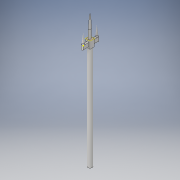
# Autodesk Inventor part: gungnir
Saved by Autodesk Inventor 2017 (Build 210142000, 142)
## iProperties
Created: 2016-12-22
Part Number: gungnir
Material: Generic
Document SubType Name: Modeling
Designer: theoren75306
Density: 1 g/cm^3
Appearance: Default
Author: theoren75306
Autodesk Inventor part; units mm, degrees
ref_plane "YZ Plane" through (0, 0, 0) normal (1, 0, 0) x (0, 1, 0)
ref_plane "XZ Plane" through (0, 0, 0) normal (0, 1, 0) x (-1, 0, 0)
ref_plane "XY Plane" through (0, 0, 0) normal (0, 0, 1) x (1, 0, 0)
sketch "Sketch1" plane through (0, 0, 0) normal (0, 1, 0) x (-1, 0, 0)
  circle A0 centre (0, 0) radius 38.1
  dimension "d0" = 76.2
  constraints: 1 centre point, 1 coincident
  measures "d0" diameter of A0
extrude "Extrusion1" add sketch "Sketch1" along normal blind 1828.8
sketch "Sketch2" plane through (0, 1828.8, 0) normal (0, 1, 0) x (1, 0, 0)
  circle A0 centre (0, 0) radius 38.1 projected
  line L0 (0, -38.1) -> (-38.1, -38.1)
  line L1 (-38.1, -38.1) -> (-38.1, 38.1)
  line L2 (-38.1, 38.1) -> (38.1, 38.1)
  line L3 (38.1, 38.1) -> (38.1, -38.1)
  line L4 (38.1, -38.1) -> (0, -38.1)
  constraints: 10 end point, 4 perpendicular, 3 horizontal, 1 point on line, 1 vertical alignment, 1 other
extrude "Extrusion2" add sketch "Sketch2" along normal blind 127 contours L0 L1 A0 | A0 L3 L4 | A0 L2 L3 | L1 L2 A0
ref_plane "Work Plane1" through (-26.9408, 1955.8, -26.9408) normal (0, 1, 0) x (1, 0, 0)
sketch "Sketch3" plane through (-26.9408, 1955.8, -26.9408) normal (0, 1, 0) x (1, 0, 0)
  circle A0 centre (26.9408, -26.9408) radius 38.1
  constraints: 1 centre point, 1 coincident
extrude "Extrusion3" add sketch "Sketch3" against normal blind 127
sketch "Sketch4" plane through (-38.1, 1828.8, 38.1) normal (0, 0, 1) x (1, 0, 0)
  line L0 (19.05, 32.3592) -> (57.15, 32.3592)
  line L1 (57.15, 32.3592) -> (57.15, 96.4699)
  line L2 (57.15, 96.4699) -> (19.05, 96.4699)
  line L3 (19.05, 96.4699) -> (19.05, 32.3592)
  arc A0 (19.05, 32.3592) -> (57.15, 32.3592) centre (38.1, 32.3592) ccw
  arc A1 (40.4667, 110.4399) -> (19.05, 96.4699) centre (53.0396, 67.7636) ccw
  arc A2 (57.15, 96.4699) -> (40.4667, 110.4399) centre (24.3533, 74.2501) ccw
  line L4 (0, 0) -> (0, 127) projected
  line L5 (76.2, 0) -> (76.2, 127) projected
  point P0 (38.1, -1828.8)
  dimension "d8" = 19.05
  dimension "d9" = 19.05
  dimension "d10" = 13.97
  constraints: 8 end point, 6 point on circle, 3 centre point, 2 parallel, 2 tangent, 1 horizontal, 1 perpendicular
  measures "d8" distance between parallel lines of L4 L3
  measures "d9" distance between parallel lines of L5 L1
  measures "d10" distance from line of L2 A1.start
extrude "Extrusion4" add sketch "Sketch4" along normal blind 101.6 contours L3 L2 L1 L0 | L0 A0
sketch "Sketch5" plane through (-38.1, 1828.8, 38.1) normal (0, 0, 1) x (1, 0, 0)
  line L0 (19.05, 32.3592) -> (19.05, 96.4699) projected
  arc A0 (38.1, 110.3729) -> (19.05, 96.4699) centre (49.9899, 74.0785) ccw
  arc A1 (56.8516, 96.4699) -> (38.1, 110.3729) centre (19.2002, 65.2848) ccw
  line L1 (19.05, 96.4699) -> (56.8516, 96.4699)
  line L2 (0, 127) -> (76.2, 127) projected
  point P0 (38.1, -1828.8)
  constraints: 4 point on circle, 2 centre point, 2 end point, 1 parallel
extrude "Extrusion5" add sketch "Sketch5" along normal blind 63.5
sketch "Sketch6" plane through (-19.05, 1925.2699, 139.7) normal (0, 1, 0) x (1, 0, 0)
  point P0 (19.05, 139.7)
sketch "Sketch7" plane through (-19.05, 1925.2699, 139.7) normal (0, 1, 0) x (1, 0, 0)
  point P0 (19.05, 139.7)
  point P1 (38.1, 0)
  point P2 (19.05, 38.1)
sketch "Sketch9" plane through (-19.05, 1925.2699, 139.7) normal (0, 1, 0) x (1, 0, 0)
  circle A0 centre (19.05, 19.0106) radius 19.05
  line L0 (38.1, 101.6) -> (38.1, 0) projected
  point P0 (19.05, 139.7)
  dimension "d25" = 38.1
  constraints: 1 centre point, 1 tangent
  measures "d25" diameter of A0
extrude "Extrusion6" add sketch "Sketch9" along normal blind 177.8
ref_plane "Work Plane4" through (38.1, 1828.8, 0) normal (0, 0, -1) x (-1, 0, 0)
mirror "Mirror1" about plane through (38.1, 1828.8, 0) normal (0, 0, -1) of "Extrusion4", "Extrusion5", "Extrusion6"
sketch "Sketch10" plane through (0, 1955.8, 0) normal (0, 1, 0) x (1, 0, 0)
  arc A0 (0, 28.3756) -> (0, -29.7598) centre (27.6643, -0.6921) ccw
  line L0 (0, -38.1) -> (-19.05, -38.1) projected
  arc A1 (0, -29.7598) -> (0, 28.3756) centre (-27.6643, -0.6921) ccw
  point P0 (0, 0)
  constraints: 4 point on circle, 2 centre point
extrude "Extrusion7" add sketch "Sketch10" along normal blind 381
chamfer "Chamfer4" distance 12.192 angle 87 2 edges at (12.4636, 2336.8, 0.6921) (-12.4636, 2336.8, 0.6921) measured on face at (11.9636, 2336.8, 0.6921) measured on face at (-11.9636, 2336.8, 0.6921)
chamfer "Chamfer5" distance 19.05 angle 83 1 edges at (-19.05, 2103.0699, 120.6894) measured on face at (-18.55, 2103.0699, 120.6894)
chamfer "Chamfer6" distance 19.05 angle 83 1 edges at (-19.05, 2103.0699, -120.6894) measured on face at (-18.55, 2103.0699, -120.6894)
body "Solid1"
